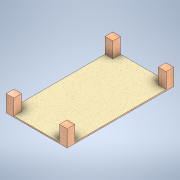
# Autodesk Inventor part: board
Saved by Autodesk Inventor 2022 (Build 260153070, 153G)
## iProperties
Created: 2021-07-07
Part Number: board
Material: Wood (Birch)
Document SubType Name: Modeling
Designer: sachin
Density: 0.55 g/cm^3
Appearance: Birch - Natural Polished
Author: sachin
Autodesk Inventor part; units mm, degrees
ref_plane "YZ Plane" through (0, 0, 0) normal (1, 0, 0) x (0, 1, 0)
ref_plane "XZ Plane" through (0, 0, 0) normal (0, 1, 0) x (-1, 0, 0)
ref_plane "XY Plane" through (0, 0, 0) normal (0, 0, 1) x (1, 0, 0)
sketch "Sketch1" plane through (0, 0, 0) normal (0, 1, 0) x (-1, 0, 0)
  line L0 (140.4432, 454.8476) -> (-259.5568, 454.8476)
  line L1 (-259.5568, 454.8476) -> (-259.5568, -245.1524)
  line L2 (-259.5568, -245.1524) -> (140.4432, -245.1524)
  line L3 (140.4432, -245.1524) -> (140.4432, 454.8476)
  point P0 (0, 0)
  dimension "d0" = 700
  dimension "d1" = 400
  constraints: 8 end point, 2 parallel, 1 horizontal, 1 perpendicular
  measures "d0" distance of L2.end L0.start
  measures "d1" distance of L1.end L2.end
extrude "Extrusion1" add sketch "Sketch1" along normal blind 8
sketch "Sketch2" plane through (0, 8, 0) normal (0, 1, 0) x (1, 0, 0)
  line L0 (-140.4432, 245.1524) -> (-140.4432, -454.8476) projected
  line L1 (-140.4432, -454.8476) -> (-89.6432, -454.8476)
  line L2 (-89.6432, -454.8476) -> (-89.6432, -404.0476)
  line L3 (-89.6432, -404.0476) -> (-140.4432, -404.0476)
  line L4 (-140.4432, -404.0476) -> (-140.4432, -454.8476)
  line L5 (259.5568, -454.8476) -> (259.5568, 245.1524) projected
  line L6 (259.5568, -454.8476) -> (208.7568, -454.8476)
  line L7 (208.7568, -454.8476) -> (208.7568, -404.0476)
  line L8 (208.7568, -404.0476) -> (259.5568, -404.0476)
  line L9 (259.5568, -404.0476) -> (259.5568, -454.8476)
  line L10 (259.5568, 245.1524) -> (208.7568, 245.1524)
  line L11 (208.7568, 245.1524) -> (208.7568, 194.3524)
  line L12 (208.7568, 194.3524) -> (259.5568, 194.3524)
  line L13 (259.5568, 194.3524) -> (259.5568, 245.1524)
  line L14 (-140.4432, 245.1524) -> (-89.6432, 245.1524)
  line L15 (-89.6432, 245.1524) -> (-89.6432, 194.3524)
  line L16 (-89.6432, 194.3524) -> (-140.4432, 194.3524)
  line L17 (-140.4432, 194.3524) -> (-140.4432, 245.1524)
  point P0 (0, 0)
  point P1 (259.5568, -404.0476)
  dimension "d4" = 50.8
  dimension "d5" = 50.8
  dimension "d6" = 50.8
  dimension "d7" = 50.8
  dimension "d8" = 50.8
  dimension "d9" = 50.8
  dimension "d10" = 50.8
  constraints: 32 end point, 8 parallel, 4 horizontal, 4 perpendicular, 1 point on line
  measures "d4" distance of L2.end L3.end
  measures "d5" distance of L1.end L2.end
  measures "d6" distance of L15.end L16.end
  measures "d7" distance of L14.end L15.end
  measures "d8" distance of L10.end L11.end
  measures "d9" distance of L11.end L12.end
  measures "d10" distance of L6.end L7.end
extrude "Extrusion2" add sketch "Sketch2" along normal blind 101.6
body "Solid1"
